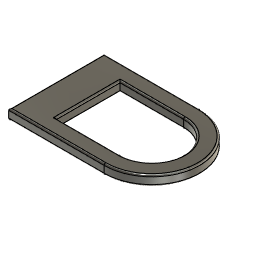
tpu-tool-hook (Autodesk Fusion 360 design; units mm, degrees)
Autodesk Fusion 360 part; units mm, degrees
sketch "Sketch1" plane through (0, 0, 0) normal (0, 0, 1) x (1, 0, 0)
  line L0 (0, 15.24) -> (45.72, 15.24)
  line L1 (45.72, 15.24) -> (45.72, -15.24)
  line L2 (45.72, -15.24) -> (0, -15.24)
  line L3 (0, -15.24) -> (0, 15.24)
  line L4 (40.64, -10.16) -> (10.16, -10.16)
  line L5 (10.16, -10.16) -> (10.16, 10.16)
  line L6 (10.16, 10.16) -> (40.64, 10.16)
  line L7 (40.64, 10.16) -> (40.64, -10.16)
  line L8 (40.64, -10.16) -> (10.16, 10.16) construction
  line L9 (10.16, -10.16) -> (40.64, 10.16) construction
  point P0 (25.4, 0)
  dimension "d1" = 45.72
  dimension "d2" = 30.48
  constraint horizontal L0
  constraint vertical L1
  constraint horizontal L2
  constraint vertical L3
  constraint horizontal L4
  constraint perpendicular L4 L5
  constraint parallel L4 L6
  constraint parallel L5 L7
  constraint coincident L8 P0
  constraint coincident L9 P0
  measures "d1" distance of L0.start L0.end
  measures "d2" distance of L0.start L2.end
extrude "Extrude1" add sketch "Sketch1" along normal blind 3.175
fillet "Fillet1" radius 10.16 2 edges at (40.64, 10.16, 1.5875) (40.64, -10.16, 1.5875)
fillet "Fillet2" radius 15.24 2 edges at (45.72, -15.24, 1.5875) (45.72, 15.24, 1.5875)
fillet "Fillet3" radius 0.508 2 faces at (3.3867, 3.3867, 3.175) (3.3867, 3.3867, 0)
